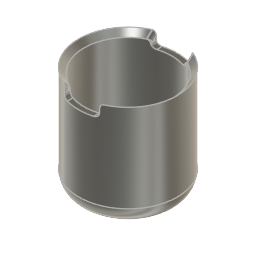
basic_potjie_finger_cutouts (Autodesk Fusion 360 design; units mm, degrees)
Autodesk Fusion 360 part; units mm, degrees
sketch "Sketch1" plane through (0, 0, 0) normal (0, 0, 1) x (1, 0, 0)
  circle A0 centre (0, 0) radius 25
  circle A1 centre (0, 0) radius 28
  dimension "d4" = 50
  dimension "d5" = 56
  constraint coincident A0.centre A1.centre
  measures "d4" diameter of A0
  measures "d5" diameter of A1
extrude "Extrude1" add sketch "Sketch1" along normal blind 3 contours A0
extrude "Extrude2" add sketch "Sketch1" along normal blind 60
fillet "Fillet1" radius 7 1 edges at (-23.3082, -9.0404, 3)
fillet "Fillet2" radius 10 1 edges at (-26.1052, -10.1252, 0)
chamfer "Chamfer1" distance 3 angle 45 1 edges at (-23.3082, 9.0404, 60)
sketch "Sketch2" plane through (0, 0, 0) normal (0, 1, 0) x (1, 0, 0)
  line L0 (0, 0) -> (0, -60)
  line L1 (0, -60) -> (10, -60)
  line L2 (10, -60) -> (-10, -60)
  line L3 (-10, -60) -> (-10, -53)
  line L4 (-10, -53) -> (10, -53)
  line L5 (10, -53) -> (10, -60)
  dimension "d18" = 60
  dimension "d20" = 10
  dimension "d21" = 20
  dimension "d22" = 7
  constraint coincident L0.start origin
  constraint vertical L0
  constraint perpendicular L0 L1
  constraint horizontal L2
  constraint vertical L3
  constraint horizontal L4
  constraint vertical L5
  measures "d18" distance of L0.start L0.end
  measures "d20" distance of L0.end L1.end
  measures "d21" distance of L1.end L2.end
  measures "d22" distance of L1.end L4.end
extrude "Extrude3" cut sketch "Sketch2" along normal blind 28
fillet "Fillet3" radius 2.5 2 edges at (10, 24.5331, 53) (-10, 24.5331, 53)
fillet "Fillet4" radius 2.5 2 edges at (10, 24.4872, 58.4504) (-10, 24.4872, 58.4504)
pattern_circular "C-Pattern1" count 2 over 360 about axis through (0, 0, 1.75) along (0, 0, 1) of "Extrude3", "Fillet3", "Fillet4"
equation "wall_thinkness = 3 mm"
equation "pot_height = 60 mm"
equation "pot_diameter = 50 mm"
equation "d4 = pot_diameter"
equation "d5 = pot_diameter + ( 2 * wall_thinkness )"
equation "d6 = wall_thinkness"
equation "d8 = pot_height"
equation "pot_bottom_outer_fillet = 10 mm"
equation "d12 = pot_bottom_outer_fillet - wall_thinkness"
equation "d14 = pot_bottom_outer_fillet"
equation "d15 = wall_thinkness"
equation "pot_finger_cutout_num = 2"
equation "pot_finger_cutout_width = 20 mm"
equation "d18 = pot_height"
equation "pot_finger_cutout_height = 7 mm"
equation "d20 = pot_finger_cutout_width / 2"
equation "d21 = pot_finger_cutout_width"
equation "d22 = pot_finger_cutout_height"
equation "d23 = ( pot_diameter + wall_thinkness * 2 ) / 2"
equation "d26 = pot_finger_cutout_height / 2 - 1 mm"
equation "d28 = pot_finger_cutout_height / 2 - 1 mm"
equation "d29 = pot_finger_cutout_num"
named bodies: "simple_potjie"
